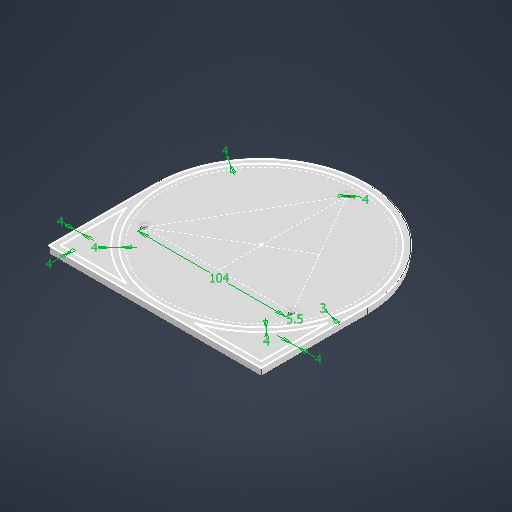
# Autodesk Inventor part: Part1
Saved by Autodesk Inventor 2026.2 (Build 302298000, 298)
## iProperties
Created: 2026-02-25
Part Number: Part1
Material: Generic
Document SubType Name: Modeling
Designer: Tathagata Sikdar
Density: 1 g/cm^3
Appearance: Default
Author: Tathagata Sikdar
Autodesk Inventor part; units mm, degrees
ref_plane "YZ Plane" through (0, 0, 0) normal (1, 0, 0) x (0, 1, 0)
ref_plane "XZ Plane" through (0, 0, 0) normal (0, 1, 0) x (-1, 0, 0)
ref_plane "XY Plane" through (0, 0, 0) normal (0, 0, 1) x (1, 0, 0)
sketch "Sketch1" plane through (0, 0, 0) normal (0, 1, 0) x (-1, 0, 0)
  line L0 (0, -60.0444) -> (52, 30.0222) construction
  line L1 (52, 30.0222) -> (-52, 30.0222) construction
  line L2 (-52, 30.0222) -> (0, -60.0444) construction
  line L3 (-26, -15.0111) -> (52, 30.0222) construction
  line L4 (0, -60.0444) -> (0, 30.0222) construction
  circle A0 centre (0, -60.0444) radius 2
  circle A1 centre (-52, 30.0222) radius 2
  circle A2 centre (52, 30.0222) radius 2
  circle A3 centre (0, 0) radius 67.5444 construction
  line L5 (74.5444, 0) -> (74.5444, 74.5444)
  line L6 (-74.5444, 0) -> (-74.5444, 74.5444)
  line L7 (74.5444, 74.5444) -> (-74.5444, 74.5444)
  line L8 (70.5444, 70.5444) -> (70.5444, 24.0906)
  line L9 (-70.5444, 24.0906) -> (-70.5444, 70.5444)
  circle A4 centre (0, 0) radius 70.5444
  arc A5 (70.5444, 24.0906) -> (24.0906, 70.5444) centre (0, 0) ccw
  arc A6 (-24.0906, 70.5444) -> (-70.5444, 24.0906) centre (0, 0) ccw
  arc A7 (-74.5444, 0) -> (74.5444, 0) centre (0, 0) ccw
  line L10 (-70.5444, 70.5444) -> (-24.0906, 70.5444)
  line L11 (24.0906, 70.5444) -> (70.5444, 70.5444)
  dimension "d0" = 4
  dimension "d1" = 104
  dimension "d2" = 5.5
  dimension "d11" = 4
  dimension "d13" = 4
  dimension "d19" = 3
  dimension "d20" = 4
  dimension "d21" = 4
  dimension "d22" = 4
  dimension "d25" = 4
  constraints: 24 end point, 8 centre point, 6 coincident, 6 point on circle, 4 perpendicular, 3 tangent, 2 equal length, 2 equal radius, 2 horizontal, 2 midpoint, 2 point on line, 2 vertical, 1 collinear, 1 concentric
  measures "d0" diameter of A0
  measures "d1" distance of L0.end L1.end
  measures "d11" distance between parallel lines of L9 L6
  measures "d13" distance between parallel lines of L5 L8
  measures "d19" radial gap between concentric circles of A3 A4
  measures "d20" radial gap between concentric circles of A7 A4
  measures "d21" radial gap between concentric circles of A4 A6
  measures "d22" radial gap between concentric circles of A4 A5
  measures "d25" distance between parallel lines of L7 L11
extrude "Extrusion2" add sketch "Sketch1" against normal blind 5 contours A7 L6 L7 L5 | L8 A5 L11 | L9 L10 A6 | A4
body "Solid2"
